metal cutting plate_v6 (Autodesk Fusion 360 design; units mm, degrees)
Autodesk Fusion 360 part; units mm, degrees
note: some values were not read from the file. Set by a fixed rule: which sketch regions a step uses.
sketch "Sketch1" plane through (0, 0, 0) normal (0, 1, 0) x (1, 0, 0)
  line L0 (82.5, 50) -> (-82.5, 50)
  line L1 (-82.5, 50) -> (-82.5, -50)
  line L2 (-82.5, -50) -> (82.5, -50)
  line L3 (82.5, -50) -> (82.5, 50)
  line L4 (82.5, 50) -> (-82.5, -50) construction
  line L5 (-82.5, 50) -> (82.5, -50) construction
  dimension "d1" = 165
  dimension "d2" = 100
  constraint horizontal L0
  constraint perpendicular L0 L1
  constraint parallel L0 L2
  constraint parallel L1 L3
  constraint coincident L4 origin
  constraint coincident L5 origin
  measures "d1" distance of L1.end L2.end
  measures "d2" distance of L0.end L1.end
extrude "Extrude1" add sketch "Sketch1" along normal blind 3 makes body 1
fillet "Fillet1" radius 10 2 edges at (82.5, 1.5, 50) (-82.5, 1.5, 50) on bodies 1
sketch "Sketch2" plane through (0, 0, 0) normal (0, -1, 0) x (1, 0, 0)
  arc A0 (-72.5, 50) -> (-82.5, 40) centre (-72.5, 40) ccw
  line L0 (-82.5, 40) -> (-82.5, -50)
  line L1 (-82.5, -50) -> (82.5, -50)
  line L2 (82.5, -50) -> (82.5, 40)
  arc A1 (82.5, 40) -> (72.5, 50) centre (72.5, 40) ccw
  line L3 (72.5, 50) -> (-72.5, 50)
  circle A2 centre (0, 10) radius 20
  circle A3 centre (-55, 30) radius 5
  circle A4 centre (55, 30) radius 5
  line L4 (-55, 30) -> (55, 30) construction
  line L5 (-72.5, -50) -> (-72.5, -296) construction
  line L6 (72.5, -50) -> (72.5, -15) construction
  circle A5 centre (-72.5, -40) radius 1.6
  circle A6 centre (-72.5, -25) radius 1.6
  circle A7 centre (72.5, -40) radius 1.6
  circle A8 centre (72.5, -25) radius 1.6
  line L7 (23.5, -13.5) -> (-23.5, -13.5)
  line L8 (-23.5, -13.5) -> (-23.5, 33.5)
  line L9 (-23.5, 33.5) -> (23.5, 33.5)
  line L10 (23.5, 33.5) -> (23.5, -13.5)
  line L11 (23.5, -13.5) -> (-23.5, 33.5) construction
  line L12 (-23.5, -13.5) -> (23.5, 33.5) construction
  circle A9 centre (-23.5, 33.5) radius 2.5
  circle A10 centre (-23.5, -13.5) radius 2.5
  circle A11 centre (23.5, -13.5) radius 2.5
  circle A12 centre (23.5, 33.5) radius 2.5
  line L13 (-47.5, 22.5) -> (-62.5, 22.5)
  line L14 (-62.5, 22.5) -> (-62.5, 37.5)
  line L15 (-62.5, 37.5) -> (-47.5, 37.5)
  line L16 (-47.5, 37.5) -> (-47.5, 22.5)
  line L17 (-47.5, 22.5) -> (-62.5, 37.5) construction
  line L18 (-62.5, 22.5) -> (-47.5, 37.5) construction
  circle A13 centre (-47.5, 37.5) radius 1.5
  circle A14 centre (-62.5, 37.5) radius 1.5
  circle A15 centre (-62.5, 22.5) radius 1.5
  circle A16 centre (-47.5, 22.5) radius 1.5
  line L19 (62.5, 22.5) -> (47.5, 22.5)
  line L20 (47.5, 22.5) -> (47.5, 37.5)
  line L21 (47.5, 37.5) -> (62.5, 37.5)
  line L22 (62.5, 37.5) -> (62.5, 22.5)
  line L23 (62.5, 22.5) -> (47.5, 37.5) construction
  line L24 (47.5, 22.5) -> (62.5, 37.5) construction
  circle A17 centre (47.5, 37.5) radius 1.5
  circle A18 centre (47.5, 22.5) radius 1.5
  circle A19 centre (62.5, 22.5) radius 1.5
  circle A20 centre (62.5, 37.5) radius 1.5
  point P0 (0, 10)
  point P1 (-55, 30)
  point P2 (55, 30)
  dimension "d7" = 40
  dimension "d8" = 60
  dimension "d9" = 10
  dimension "d10" = 10
  dimension "d11" = 110
  dimension "d13" = 27.5
  dimension "d14" = 27.5
  dimension "d15" = 20
  dimension "d16" = 10
  dimension "d17" = 10
  dimension "d18" = 3.2
  dimension "d19" = 3.2
  dimension "d20" = 10
  dimension "d21" = 15
  dimension "d22" = 3.2
  dimension "d23" = 3.2
  dimension "d24" = 10
  dimension "d25" = 15
  dimension "d26" = 47
  dimension "d27" = 47
  dimension "d28" = 5
  dimension "d29" = 5
  dimension "d30" = 5
  dimension "d31" = 5
  dimension "d32" = 15
  dimension "d33" = 15
  dimension "d34" = 3
  dimension "d35" = 3
  dimension "d36" = 3
  dimension "d37" = 3
  dimension "d38" = 15
  dimension "d39" = 15
  dimension "d40" = 3
  dimension "d41" = 3
  dimension "d42" = 3
  dimension "d43" = 3
  constraint coincident P1 A3.centre
  constraint coincident P2 A4.centre
  constraint horizontal L4
  constraint coincident L1 L5.start
  constraint perpendicular L1 L5
  constraint coincident L1 L6.start
  constraint perpendicular L1 L6
  constraint coincident L5 A5.centre
  constraint coincident L5 A6.centre
  constraint coincident L6 A7.centre
  constraint coincident L6 A8.centre
  constraint horizontal L7
  constraint perpendicular L7 L8
  constraint parallel L7 L9
  constraint parallel L8 L10
  constraint coincident L11 P0
  constraint coincident L12 P0
  constraint coincident P0 A2.centre
  constraint coincident L8.end L9.start
  constraint coincident L7.end L8.start
  constraint coincident L7.start L10.end
  constraint coincident L9.end L10.start
  constraint horizontal L13
  constraint perpendicular L13 L14
  constraint parallel L13 L15
  constraint parallel L14 L16
  constraint coincident L17 P1
  constraint coincident L18 P1
  constraint coincident L15.end L16.start
  constraint coincident L14.end L15.start
  constraint coincident L13.end L14.start
  constraint coincident L13.start L16.end
  constraint horizontal L19
  constraint perpendicular L19 L20
  constraint parallel L19 L21
  constraint parallel L20 L22
  constraint coincident L23 P2
  constraint coincident L24 P2
  constraint coincident L20.end L21.start
  constraint coincident L19.end L20.start
  constraint coincident L19.start L22.end
  constraint coincident L21.end L22.start
  measures "d7" diameter of A2
  measures "d8" distance of L1 P0
  measures "d9" diameter of A3
  measures "d10" diameter of A4
  measures "d11" distance of P1 P2
  measures "d13" distance of L2 P2
  measures "d14" distance of L0 P1
  measures "d15" distance of P0 L4
  measures "d16" distance of L2 L6
  measures "d17" distance of L0 L5
  measures "d18" diameter of A5
  measures "d19" diameter of A6
  measures "d20" distance of L5.start A5.centre
  measures "d21" distance of A5.centre A6.centre
  measures "d22" diameter of A7
  measures "d23" diameter of A8
  measures "d24" distance of L1 A7.centre
  measures "d25" distance of A7.centre A8.centre
  measures "d26" distance of L8.end L9.end
  measures "d27" distance of L7.end L8.end
  measures "d28" diameter of A9
  measures "d29" diameter of A10
  measures "d30" diameter of A11
  measures "d31" diameter of A12
  measures "d32" distance of L14.end L15.end
  measures "d33" distance of L13.end L14.end
  measures "d34" diameter of A13
  measures "d35" diameter of A14
  measures "d36" diameter of A15
  measures "d37" diameter of A16
  measures "d38" distance of L20.end L21.end
  measures "d39" distance of L19.end L20.end
  measures "d40" diameter of A17
  measures "d41" diameter of A18
  measures "d42" diameter of A19
  measures "d43" diameter of A20
extrude "Extrude2" cut sketch "Sketch2" against normal blind 10 contours A2 | A3 | A4 | A5 | A6 | A7 | A8 | L7 L8 A10 | L7 L8 A10 | L7 L10 A11 | L7 L10 A11 | L8 L9 A9 | L8 L9 A9 | L9 L10 A12 | L9 L10 A12 | L13 L14 A15 | L13 L14 A15 | L13 L16 A16 | L13 L16 A16 | L14 L15 A14 | L14 L15 A14 | L15 L16 A13 | L15 L16 A13 | L19 L20 A18 | L19 L20 A18 | L19 L22 A19 | L19 L22 A19 | L20 L21 A17 | L20 L21 A17 | L21 L22 A20 | L21 L22 A20 bodies 1
ref_plane "WorkPlane1" through (0, 0, 0) normal (0, -1, 0) x (-1, 0, 0)
sketch "Sketch3" plane through (0, 0, 0) normal (0, -1, 0) x (1, 0, 0)
  line L0 (67.5, 17.5) -> (42.5, 17.5)
  line L1 (42.5, 17.5) -> (42.5, 42.5)
  line L2 (42.5, 42.5) -> (67.5, 42.5)
  line L3 (67.5, 42.5) -> (67.5, 17.5)
  line L4 (67.5, 17.5) -> (42.5, 42.5) construction
  line L5 (42.5, 17.5) -> (67.5, 42.5) construction
  circle A0 centre (47.5, 37.5) radius 1.5
  circle A1 centre (62.5, 37.5) radius 1.5
  circle A2 centre (62.4953, 22.5047) radius 1.5
  circle A3 centre (47.5, 22.5) radius 1.5
  circle A4 centre (55, 30) radius 5
  circle A5 centre (55, 30) radius 6.25
  point P0 (55, 30)
  dimension "d47" = 25
  dimension "d48" = 25
  dimension "d49" = 3
  dimension "d50" = 3
  dimension "d51" = 3
  dimension "d52" = 3
  dimension "d53" = 10
  dimension "d54" = 12.5
  constraint horizontal L0
  constraint perpendicular L0 L1
  constraint parallel L0 L2
  constraint parallel L1 L3
  constraint coincident L4 P0
  constraint coincident L5 P0
  constraint coincident L4 A0.centre
  constraint coincident L5 A1.centre
  constraint coincident L4 A2.centre
  constraint coincident L5 A3.centre
  constraint coincident P0 A4.centre
  constraint concentric A4 A5
  measures "d47" distance of L1.end L2.end
  measures "d48" distance of L0.end L1.end
  measures "d49" diameter of A0
  measures "d50" diameter of A1
  measures "d51" diameter of A2
  measures "d52" diameter of A3
  measures "d53" diameter of A4
  measures "d54" diameter of A5
extrude "Extrude1'" add sketch "Sketch3" along normal blind 5 separate body contours L0 L1 L2 L3 makes body 2 in component "Component"
extrude "Extrude2'" add sketch "Sketch3" along normal blind 15 contours A5 bodies 2 in component "Component"
sketch "Sketch4" plane through (0, -15, 0) normal (0, -1, 0) x (1, 0, 0)
  circle A0 centre (55, 30) radius 5
  circle A1 centre (55, 30) radius 6.25
  circle A2 centre (55, 30) radius 6.25
  constraint concentric A0 A2
extrude "Extrude3" add sketch "Sketch4" along normal blind 2.5 contours A0 | A1 A2 bodies 2 in component "Component"
fillet "Fillet1'" radius 2.5 1 edges at (49.173, -5, 32.2601) on bodies 2 in component "Component"
fillet "Fillet2" radius 1 8 edges at (55, -5, 17.5) (42.5, -5, 30) (55, -5, 42.5) (67.5, -5, 30) (42.5, -2.5, 17.5) (67.5, -2.5, 17.5) (42.5, -2.5, 42.5) (67.5, -2.5, 42.5) on bodies 2 in component "Component"
fillet "Fillet3" radius 0.5 1 edges at (49.173, -17.5, 27.7399) on bodies 2 in component "Component"
sketch "Sketch5" plane through (0, 0.4541, 0) normal (0, -1, 0) x (1, 0, 0)
  circle A0 centre (121.9573, 29.9908) radius 8.75
  circle A1 centre (129.4526, 22.4955) radius 1.5
  circle A2 centre (114.4573, 37.4908) radius 1.5
  circle A3 centre (114.4573, 22.4908) radius 1.5
  circle A4 centre (129.4573, 37.4908) radius 1.5
  line L0 (133.4573, 18.4908) -> (133.4573, 41.4908)
  line L1 (133.4573, 41.4908) -> (110.4573, 41.4908)
  line L2 (110.4573, 41.4908) -> (110.4573, 18.4908)
  line L3 (110.4573, 18.4908) -> (133.4573, 18.4908)
  circle A5 centre (114.4573, 37.4908) radius 2.25
  circle A6 centre (114.4573, 22.4908) radius 2.25
  circle A7 centre (129.4526, 22.4955) radius 2.25
  circle A8 centre (129.4573, 37.4908) radius 2.25
  dimension "d67" = 4.5
  dimension "d68" = 4.5
  dimension "d69" = 4.5
  dimension "d70" = 4.5
  constraint concentric A2 A5
  constraint concentric A3 A6
  constraint concentric A1 A7
  constraint concentric A4 A8
  measures "d67" diameter of A5
  measures "d68" diameter of A6
  measures "d69" diameter of A7
  measures "d70" diameter of A8
extrude "Extrude4" cut sketch "Sketch5" along normal blind 1 and the other way blind 1 contours A0 A8 | A0 A8 | A0 A7 | A0 A7 | A0 A5 | A0 A5 | A0 A6 | A0 A6 sketch seen with x (1, 0, 0) y (0, 1, 0) z (0, 0, 1) at (-66.9573, -5.4541, 0.0092) bodies 2 in component "Component"
sketch "Sketch6" plane through (0, 0, 0) normal (0, -1, 0) x (1, 0, 0)
  circle A0 centre (47.5, 37.5) radius 1.5
  circle A1 centre (-47.5, 22.5) radius 1.5
  circle A2 centre (-23.5, 33.5) radius 2.5
  circle A3 centre (72.5, -40) radius 1.6
  circle A4 centre (55, 30) radius 5
  circle A5 centre (72.5, -25) radius 1.6
  circle A6 centre (-23.5, -13.5) radius 2.5
  circle A7 centre (-62.5, 22.5) radius 1.5
  circle A8 centre (62.5, 37.5) radius 1.5
  circle A9 centre (47.5, 22.5) radius 1.5
  circle A10 centre (-47.5, 37.5) radius 1.5
  circle A11 centre (23.5, 33.5) radius 2.5
  circle A12 centre (-72.5, -40) radius 1.6
  circle A13 centre (0, 10) radius 20
  circle A14 centre (-55, 30) radius 5
  circle A15 centre (-72.5, -25) radius 1.6
  circle A16 centre (23.5, -13.5) radius 2.5
  circle A17 centre (-62.5, 37.5) radius 1.5
  circle A18 centre (62.5, 22.5) radius 1.5
  arc A19 (-72.5, 50) -> (-82.5, 40) centre (-72.5, 40) ccw
  line L0 (-82.5, 40) -> (-82.5, -50)
  line L1 (-82.5, -50) -> (82.5, -50)
  line L2 (82.5, -50) -> (82.5, 40)
  arc A20 (82.5, 40) -> (72.5, 50) centre (72.5, 40) ccw
  line L3 (72.5, 50) -> (-72.5, 50)
sketch "Sketch1 (2)" plane through (0, 0, 0) normal (0, 1, 0) x (1, 0, 0) in component "part_for_attach"
  circle A0 centre (0, 0) radius 5
  circle A1 centre (0, 0) radius 4
  dimension "d75" = 10
  dimension "d76" = 8
  constraint coincident A0.centre A1.centre
  measures "d75" diameter of A0
  measures "d76" diameter of A1
extrude "Extrude1''" add sketch "Sketch1 (2)" along normal blind 25 separate body makes body 3 in component "part_for_attach"
coil "CoilPrimitive1" add diameter 8 section square size 1 inside turns 12.5 pitch 2 right hand placed x (1, 0, 0) y (0, 0, -1) z (0, 1, 0) at (0, 0, 0) bodies 3 in component "part_for_attach"
sketch "Sketch7" plane through (0, 0, 0) normal (0, -1, 0) x (1, 0, 0)
  line L0 (30, -20) -> (-30, -20)
  line L1 (-30, -20) -> (-30, 40)
  line L2 (-30, 40) -> (30, 40)
  line L3 (30, 40) -> (30, -20)
  line L4 (30, -20) -> (-30, 40) construction
  line L5 (-30, -20) -> (30, 40) construction
  circle A0 centre (-23.4818, 33.4818) radius 2.5
  circle A1 centre (23.4542, 33.4542) radius 2.5
  circle A2 centre (-23.5534, -13.5534) radius 2.5
  circle A3 centre (23.4995, -13.4995) radius 2.5
  circle A4 centre (0, 10) radius 20
  circle A5 centre (0, 10) radius 9.5
  point P0 (0, 10)
  dimension "d84" = 60
  dimension "d85" = 60
  dimension "d86" = 5
  dimension "d87" = 5
  dimension "d88" = 5
  dimension "d89" = 5
  dimension "d90" = 40
  dimension "d91" = 19
  constraint horizontal L0
  constraint perpendicular L0 L1
  constraint parallel L0 L2
  constraint parallel L1 L3
  constraint coincident L4 P0
  constraint coincident L5 P0
  constraint coincident L4 A0.centre
  constraint coincident L5 A1.centre
  constraint coincident L5 A2.centre
  constraint coincident L4 A3.centre
  constraint coincident P0 A4.centre
  measures "d84" distance of L1.end L2.end
  measures "d85" distance of L0.end L1.end
  measures "d86" diameter of A0
  measures "d87" diameter of A1
  measures "d88" diameter of A2
  measures "d89" diameter of A3
  measures "d90" diameter of A4
  measures "d91" diameter of A5
extrude "Extrude3'" add sketch "Sketch7" along normal blind 10 separate body contours L0 L1 L2 L3 | A4 makes body 4
extrude "Extrude1'''" add sketch "Sketch7" along normal blind 10 separate body contours L0 L1 L2 L3 | A4 makes body 5 in component "Component'"
extrude "Extrude2''" add sketch "Sketch7" against normal blind 3 contours A4 bodies 5 in component "Component'"
sketch "Sketch8" plane through (0, -10, 0) normal (0, -1, 0) x (1, 0, 0)
  circle A0 centre (23.4995, -13.4995) radius 2.5
  circle A1 centre (0, 10) radius 9.5
  circle A2 centre (-23.5534, -13.5534) radius 2.5
  circle A3 centre (23.4542, 33.4542) radius 2.5
  circle A4 centre (-23.4818, 33.4818) radius 2.5
  line L0 (30, 40) -> (-30, 40)
  line L1 (-30, 40) -> (-30, -20)
  line L2 (-30, -20) -> (30, -20)
  line L3 (30, -20) -> (30, 40)
  circle A5 centre (0, 10) radius 5
  dimension "d98" = 10
  constraint concentric A1 A5
  measures "d98" diameter of A5
extrude "Extrude3''" add sketch "Sketch8" against normal blind 7 contours A1 bodies 5 in component "Component'"
delete_face "DeleteFace1" 1 faces at (63.2467, -5.0143, 28.0118) on bodies 2 in component "Component"
extrude "Extrude1''''" add sketch "Sketch3" along normal blind 20 separate body contours L0 L1 L2 L3 | A5 makes body 6 in component "Component''"
sketch "Sketch9" plane through (0, 158.9934, 0) normal (0, -1, 0) x (1, 0, 0)
  circle A0 centre (4.4661, 94.4203) radius 1.5
  circle A1 centre (4.4614, 79.425) radius 1.5
  circle A2 centre (-10.5339, 94.4203) radius 1.5
  circle A3 centre (-10.5339, 79.4203) radius 1.5
  circle A4 centre (-3.0339, 86.9203) radius 5
  line L0 (9.4661, 99.4203) -> (-15.5339, 99.4203)
  line L1 (-15.5339, 99.4203) -> (-15.5339, 74.4203)
  line L2 (-15.5339, 74.4203) -> (9.4661, 74.4203)
  line L3 (9.4661, 74.4203) -> (9.4661, 99.4203)
  circle A5 centre (4.4661, 94.4203) radius 3.75
  circle A6 centre (-10.5339, 94.4203) radius 3.75
  circle A7 centre (-10.5339, 79.4203) radius 3.75
  circle A8 centre (4.4614, 79.425) radius 3.75
  circle A9 centre (-3.0339, 86.9203) radius 5
  dimension "d103" = 7.5
  dimension "d104" = 7.5
  dimension "d105" = 7.5
  dimension "d106" = 7.5
  dimension "d109" = 10
  constraint concentric A0 A5
  constraint concentric A2 A6
  constraint concentric A3 A7
  constraint concentric A1 A8
  constraint concentric A4 A9
  measures "d103" diameter of A5
  measures "d104" diameter of A6
  measures "d105" diameter of A7
  measures "d106" diameter of A8
  measures "d109" diameter of A9
extrude "Extrude2'''" cut sketch "Sketch9" against normal blind 5 contours A5 | A6 | A7 | A8 sketch seen with x (1, 0, 0) y (0, 1, 0) z (0, 0, 1) at (58.0339, -178.9934, -56.9203) bodies 6 in component "Component''"
extrude "Extrude3'''" add sketch "Sketch9" against normal blind 5 contours A4 A9 sketch seen with x (1, 0, 0) y (0, 1, 0) z (0, 0, 1) at (58.0339, -178.9934, -56.9203) bodies 6 in component "Component''"
component "Component" placed x (1, 0, 0) y (0, 1, 0) z (0, 0, 1) at (66.9573, 5.4541, -0.0092)
component "part_for_attach" placed x (1, 0, 0) y (0, 1, 0) z (0, 0, 1) at (28.3888, 93.6629, -22.2467)
component "Component'" placed x (1, 0, 0) y (0, 1, 0) z (0, 0, 1) at (0, 0, 0)
component "Component''" placed x (1, 0, 0) y (0, 1, 0) z (0, 0, 1) at (-58.0339, 178.9934, 56.9203)
